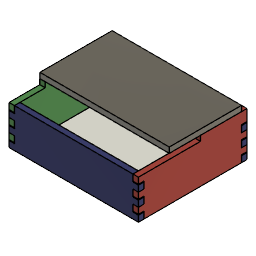
UselessBoxCardboard_v4 (Autodesk Fusion 360 design; units mm, degrees)
Autodesk Fusion 360 part; units mm, degrees
note: some values were not read from the file. Chosen so that the rebuilt part matches the saved one: a direction.
sketch "Sketch1" plane through (0, 0, 0) normal (0, 0, 1) x (1, 0, 0) in component "bottom panel"
  line L0 (0, 0) -> (91, 0)
  line L1 (91, 0) -> (91, 75)
  line L2 (91, 75) -> (0, 75)
  line L3 (0, 75) -> (0, 0)
  dimension "d116" = 75
  dimension "d117" = 91
  constraint horizontal L0
  constraint vertical L1
  constraint horizontal L2
  constraint vertical L3
  constraint coincident L0.start L3.end
  measures "d116" distance of L0.start L2.end
  measures "d117" distance of L1.end L2.end
extrude "Extrude1" add sketch "Sketch1" against normal blind 4.2 makes body 1 in component "bottom panel"
sketch "Sketch1 (2)" plane through (0, 0, 0) normal (0, -1, 0) x (1, 0, 0) in component "front panel"
  line L0 (91, 0) -> (0, 0)
  line L1 (0, 0) -> (0, -4.2)
  line L2 (0, -4.2) -> (91, -4.2)
  line L3 (91, -4.2) -> (91, 0)
  line L4 (0, 30) -> (91, 30)
  line L5 (91, 30) -> (91, 0)
  line L6 (91, 0) -> (0, 0)
  line L7 (0, 0) -> (0, 30)
  line L8 (0, 0) -> (-4.2, 0)
  line L9 (-4.2, 0) -> (-4.2, 5.3)
  line L10 (-4.2, 5.3) -> (0, 5.3)
  line L11 (0, 5.3) -> (0, 0)
  line L12 (45.5, 30) -> (45.5, 0) construction
  line L13 (95.2, 5.3) -> (91, 5.3)
  line L14 (95.2, 0) -> (95.2, 5.3)
  line L15 (91, 0) -> (95.2, 0)
  line L16 (-4.2, 15.3) -> (0, 15.3)
  line L17 (-4.2, 10) -> (-4.2, 15.3)
  line L18 (0, 10) -> (-4.2, 10)
  line L19 (-4.2, 25.3) -> (0, 25.3)
  line L20 (-4.2, 20) -> (-4.2, 25.3)
  line L21 (0, 20) -> (-4.2, 20)
  line L22 (95.2, 15.3) -> (91, 15.3)
  line L23 (95.2, 10) -> (95.2, 15.3)
  line L24 (91, 10) -> (95.2, 10)
  line L25 (95.2, 25.3) -> (91, 25.3)
  line L26 (95.2, 20) -> (95.2, 25.3)
  line L27 (91, 20) -> (95.2, 20)
  dimension "d120" = 30
  dimension "d121" = 5.3
  dimension "d123" = 4.2
  dimension "d126" = 0
  dimension "d127" = 10
  dimension "d130" = 0
  dimension "d131" = 10
  constraint horizontal L4
  constraint vertical L5
  constraint horizontal L6
  constraint vertical L7
  constraint midpoint L0 L6
  constraint equal L0 L6
  constraint horizontal L8
  constraint vertical L9
  constraint horizontal L10
  constraint vertical L11
  constraint midpoint L4 L12.start
  constraint midpoint L6 L12.end
  constraint symmetric L0.end L12 L0.start
  constraint symmetric L8.end L12 L14.start
  constraint symmetric L9.end L12 L13.start
  constraint symmetric L10.end L12 L13.end
  measures "d120" distance of L4.end L0.start
  measures "d121" distance of L8.end L9.end
  measures "d123" distance of L9.end L10.end
extrude "Extrude1'" add sketch "Sketch1 (2)" along normal blind 4.2 separate body contours L0 L4 L5 L6 L7 L11 | L5 L13 L14 L15 | L7 L8 L9 L10 L11 | L5 L22 L23 L24 | L7 L16 L17 L18 | L5 L25 L26 L27 | L7 L19 L20 L21 makes body 2 in component "front panel"
sketch "Sketch1 (3)" plane through (0, 0, 0) normal (-1, 0, 0) x (0, -1, 0) in component "left panel"
  line L0 (0, 0) -> (-75, 0)
  line L1 (-75, 0) -> (-75, -4.2)
  line L2 (-75, -4.2) -> (0, -4.2)
  line L3 (0, -4.2) -> (0, 0)
  line L4 (0, 0) -> (-75, 0)
  line L5 (-75, 0) -> (-75, 30)
  line L6 (-75, 30) -> (0, 30)
  line L7 (0, 30) -> (0, 0)
  line L8 (0, 10) -> (4.2, 10)
  line L9 (4.2, 10) -> (4.2, 4.7)
  line L10 (4.2, 4.7) -> (0, 4.7)
  line L11 (0, 4.7) -> (0, 10)
  line L12 (-37.5, 30) -> (-37.5, 0) construction
  line L13 (-75, 10) -> (-79.2, 10)
  line L14 (-79.2, 10) -> (-79.2, 4.7)
  line L15 (-79.2, 4.7) -> (-75, 4.7)
  line L16 (4.2, 14.7) -> (0, 14.7)
  line L17 (4.2, 20) -> (4.2, 14.7)
  line L18 (0, 20) -> (4.2, 20)
  line L19 (4.2, 24.7) -> (0, 24.7)
  line L20 (4.2, 30) -> (4.2, 24.7)
  line L21 (0, 30) -> (4.2, 30)
  line L22 (-75, 20) -> (-79.2, 20)
  line L23 (-79.2, 20) -> (-79.2, 14.7)
  line L24 (-79.2, 14.7) -> (-75, 14.7)
  line L25 (-75, 30) -> (-79.2, 30)
  line L26 (-79.2, 30) -> (-79.2, 24.7)
  line L27 (-79.2, 24.7) -> (-75, 24.7)
  dimension "d134" = 75
  dimension "d135" = 30
  dimension "d136" = 4.2
  dimension "d137" = 5.3
  dimension "d138" = 4.7
  dimension "d141" = 0
  dimension "d142" = 10
  dimension "d145" = 0
  dimension "d146" = 10
  constraint horizontal L4
  constraint vertical L5
  constraint horizontal L6
  constraint vertical L7
  constraint coincident L0.start L3.end
  constraint horizontal L8
  constraint vertical L9
  constraint horizontal L10
  constraint vertical L11
  constraint coincident L7 L8.start
  constraint midpoint L6 L12.start
  constraint midpoint L4 L12.end
  constraint symmetric L8.start L12 L13.start
  constraint symmetric L8.end L12 L13.end
  constraint symmetric L9.end L12 L14.end
  constraint symmetric L10.end L12 L15.end
  measures "d134" distance of L5.end L6.end
  measures "d135" distance of L0.end L5.end
  measures "d136" distance of L8.start L8.end
  measures "d137" distance of L8.end L9.end
  measures "d138" distance of L0.start L10
extrude "Extrude1''" add sketch "Sketch1 (3)" along normal blind 4.2 separate body contours L0 L4 L5 L6 L7 L11 | L7 L8 L9 L10 L11 | L5 L13 L14 L15 | L7 L16 L17 L18 | L5 L22 L23 L24 | L7 L19 L20 L21 | L5 L25 L26 L27 makes body 3 in component "left panel"
ref_plane "WorkPlane1" through (45.5, 37.5, -2.1) normal (-1, 0, 0) x (0, 1, 0)
ref_plane "WorkPlane2" through (45.5, 37.5, -2.1) normal (0, -1, 0) x (-1, 0, 0)
mirror "MirrorComponent1" about plane through (0, 0, 0) normal (0, 0, 1) of bodies 3 makes body 4 in component "right panel"
mirror "MirrorComponent2" about plane through (0, 0, 0) normal (0, 0, 1) of bodies 2 makes body 5 in component "back panel"
sketch "Sketch15" plane through (0, 0, 30) normal (0, 0, 1) x (-1, 0, 0)
  line L0 (0, 4.2) -> (0, -79.2)
  line L1 (0, -79.2) -> (4.2, -79.2)
  line L2 (4.2, -79.2) -> (4.2, 4.2)
  line L3 (4.2, 4.2) -> (0, 4.2)
  line L4 (0, 4.2) -> (4.2, 4.2)
  line L5 (4.2, 4.2) -> (4.2, -19.45)
  line L6 (4.2, -19.45) -> (0, -19.45)
  line L7 (0, -19.45) -> (0, 4.2)
  dimension "d213" = 4.2
  dimension "d214" = 23.65
  constraint horizontal L4
  constraint vertical L5
  constraint horizontal L6
  constraint vertical L7
  constraint coincident L0.start L3.end
  measures "d213" distance of L0.start L2.end
  measures "d214" distance of L0.start L6.end
extrude "Extrude3" add sketch "Sketch15" along normal blind 4 contours L0 L1 L2 L6 bodies 3 in component "left panel"
extrude "Extrude1'''" add 1 faces at (30.3333, -1.4, -30) along direction (0, 0, -1) blind 4 on bodies 5 bodies 5 in component "back panel"
sketch "Sketch16" plane through (0, 0, 30) normal (0, 0, 1) x (-1, 0, 0)
  line L0 (-91, -79.2) -> (-91, 4.2)
  line L1 (-91, 4.2) -> (-95.2, 4.2)
  line L2 (-95.2, 4.2) -> (-95.2, -79.2)
  line L3 (-95.2, -79.2) -> (-91, -79.2)
  line L4 (-95.2, 4.2) -> (-91, 4.2)
  line L5 (-91, 4.2) -> (-91, -43.45)
  line L6 (-91, -43.45) -> (-95.2, -43.45)
  line L7 (-95.2, -43.45) -> (-95.2, 4.2)
  dimension "d219" = 4.2
  dimension "d220" = 47.65
  constraint horizontal L4
  constraint vertical L5
  constraint horizontal L6
  constraint vertical L7
  constraint coincident L1.end L2.start
  measures "d219" distance of L1.end L0.end
  measures "d220" distance of L1.end L6.end
extrude "Extrude2" add sketch "Sketch16" along normal blind 4 contours L0 L2 L3 L6 sketch seen with x (-1, 0, 0) y (0, 1, 0) z (0, 0, -1) at (91, 0, 0) bodies 4 in component "right panel"
sketch "Sketch2" plane through (0, 0, 34) normal (0, 0, 1) x (-1, 0, 0) in component "lid"
  line L0 (4.2, -19.45) -> (0, -19.45)
  line L1 (0, -19.45) -> (0, -79.2)
  line L2 (0, -79.2) -> (4.2, -79.2)
  line L3 (4.2, -79.2) -> (4.2, -19.45)
  line L4 (4.2, -79.2) -> (-95.2, -79.2)
  line L5 (-95.2, -79.2) -> (-95.2, -19.2)
  line L6 (-95.2, -19.2) -> (4.2, -19.2)
  line L7 (4.2, -19.2) -> (4.2, -79.2)
  dimension "d225" = 99.4
  dimension "d226" = 60
  constraint horizontal L4
  constraint vertical L5
  constraint horizontal L6
  constraint vertical L7
  constraint coincident L2.end L3.start
  measures "d225" distance of L2.end L4.end
  measures "d226" distance of L2.end L6.end
extrude "Extrude2'" add sketch "Sketch2" along normal blind 4.2 separate body makes body 6 in component "lid"
move_face "OffsetFaces1" offset -4.5 1 faces at (28.9333, 19.2, 35.4) on bodies 6 in component "lid"
sketch "Sketch18" plane through (0, 0, 0) normal (0, 0, 1) x (-1, 0, 0)
  line L0 (-95.2, -164.5) -> (4.2, -164.5)
  line L1 (4.2, -164.5) -> (4.2, -109)
  line L2 (4.2, -109) -> (-95.2, -109)
  line L3 (-95.2, -109) -> (-95.2, -164.5)
  line L4 (-91, -85) -> (-95.2, -85)
  line L5 (-95.2, -85) -> (-95.2, -90.3)
  line L6 (-95.2, -90.3) -> (-91, -90.3)
  line L7 (-91, -90.3) -> (-91, -95)
  line L8 (-91, -95) -> (-95.2, -95)
  line L9 (-95.2, -95) -> (-95.2, -100.3)
  line L10 (-95.2, -100.3) -> (-91, -100.3)
  line L11 (-91, -100.3) -> (-91, -109)
  line L12 (-91, -109) -> (0, -109)
  line L13 (0, -109) -> (0, -100.3)
  line L14 (0, -100.3) -> (4.2, -100.3)
  line L15 (4.2, -100.3) -> (4.2, -95)
  line L16 (4.2, -95) -> (0, -95)
  line L17 (0, -95) -> (0, -90.3)
  line L18 (0, -90.3) -> (4.2, -90.3)
  line L19 (4.2, -90.3) -> (4.2, -85)
  line L20 (4.2, -85) -> (0, -85)
  line L21 (0, -85) -> (0, -80.3)
  line L22 (0, -80.3) -> (4.2, -80.3)
  line L23 (4.2, -80.3) -> (4.2, -75)
  line L24 (4.2, -75) -> (-95.2, -75)
  line L25 (-95.2, -75) -> (-95.2, -80.3)
  line L26 (-95.2, -80.3) -> (-91, -80.3)
  line L27 (-91, -80.3) -> (-91, -85)
  line L28 (0, -75) -> (0, 0)
  line L29 (0, 0) -> (-91, 0)
  line L30 (-91, 0) -> (-91, -75)
  line L31 (-91, -75) -> (0, -75)
  line L32 (30, -19.45) -> (30, 4.2)
  line L33 (30, 4.2) -> (24.7, 4.2)
  line L34 (24.7, 4.2) -> (24.7, 0)
  line L35 (24.7, 0) -> (20, 0)
  line L36 (20, 0) -> (20, 4.2)
  line L37 (20, 4.2) -> (14.7, 4.2)
  line L38 (14.7, 4.2) -> (14.7, 0)
  line L39 (14.7, 0) -> (10, 0)
  line L40 (10, 0) -> (10, 4.2)
  line L41 (10, 4.2) -> (4.7, 4.2)
  line L42 (4.7, 4.2) -> (4.7, 0)
  line L43 (4.7, 0) -> (0, 0)
  line L44 (0, 0) -> (0, -75)
  line L45 (0, -75) -> (4.7, -75)
  line L46 (4.7, -75) -> (4.7, -79.2)
  line L47 (4.7, -79.2) -> (10, -79.2)
  line L48 (10, -79.2) -> (10, -75)
  line L49 (10, -75) -> (14.7, -75)
  line L50 (14.7, -75) -> (14.7, -79.2)
  line L51 (14.7, -79.2) -> (20, -79.2)
  line L52 (20, -79.2) -> (20, -75)
  line L53 (20, -75) -> (24.7, -75)
  line L54 (24.7, -75) -> (24.7, -79.2)
  line L55 (24.7, -79.2) -> (34, -79.2)
  line L56 (34, -79.2) -> (34, -19.45)
  line L57 (34, -19.45) -> (30, -19.45)
  line L58 (-95.2, 10) -> (-91, 10)
  line L59 (-91, 10) -> (-91, 5.3)
  line L60 (-91, 5.3) -> (-95.2, 5.3)
  line L61 (-95.2, 5.3) -> (-95.2, 0)
  line L62 (-95.2, 0) -> (4.2, 0)
  line L63 (4.2, 0) -> (4.2, 5.3)
  line L64 (4.2, 5.3) -> (0, 5.3)
  line L65 (0, 5.3) -> (0, 10)
  line L66 (0, 10) -> (4.2, 10)
  line L67 (4.2, 10) -> (4.2, 15.3)
  line L68 (4.2, 15.3) -> (0, 15.3)
  line L69 (0, 15.3) -> (0, 20)
  line L70 (0, 20) -> (4.2, 20)
  line L71 (4.2, 20) -> (4.2, 25.3)
  line L72 (4.2, 25.3) -> (0, 25.3)
  line L73 (0, 25.3) -> (0, 30)
  line L74 (0, 30) -> (-91, 30)
  line L75 (-91, 30) -> (-91, 25.3)
  line L76 (-91, 25.3) -> (-95.2, 25.3)
  line L77 (-95.2, 25.3) -> (-95.2, 20)
  line L78 (-95.2, 20) -> (-91, 20)
  line L79 (-91, 20) -> (-91, 15.3)
  line L80 (-91, 15.3) -> (-95.2, 15.3)
  line L81 (-95.2, 15.3) -> (-95.2, 10)
  line L82 (-125, -79.2) -> (-115.7, -79.2)
  line L83 (-115.7, -79.2) -> (-115.7, -75)
  line L84 (-115.7, -75) -> (-111, -75)
  line L85 (-111, -75) -> (-111, -79.2)
  line L86 (-111, -79.2) -> (-105.7, -79.2)
  line L87 (-105.7, -79.2) -> (-105.7, -75)
  line L88 (-105.7, -75) -> (-101, -75)
  line L89 (-101, -75) -> (-101, -79.2)
  line L90 (-101, -79.2) -> (-95.7, -79.2)
  line L91 (-95.7, -79.2) -> (-95.7, -75)
  line L92 (-95.7, -75) -> (-91, -75)
  line L93 (-91, -75) -> (-91, 0)
  line L94 (-91, 0) -> (-95.7, 0)
  line L95 (-95.7, 0) -> (-95.7, 4.2)
  line L96 (-95.7, 4.2) -> (-101, 4.2)
  line L97 (-101, 4.2) -> (-101, 0)
  line L98 (-101, 0) -> (-105.7, 0)
  line L99 (-105.7, 0) -> (-105.7, 4.2)
  line L100 (-105.7, 4.2) -> (-111, 4.2)
  line L101 (-111, 4.2) -> (-111, 0)
  line L102 (-111, 0) -> (-115.7, 0)
  line L103 (-115.7, 0) -> (-115.7, 4.2)
  line L104 (-115.7, 4.2) -> (-121, 4.2)
  line L105 (-121, 4.2) -> (-121, -43.45)
  line L106 (-121, -43.45) -> (-125, -43.45)
  line L107 (-125, -43.45) -> (-125, -79.2)
component "bottom panel" placed x (1, 0, 0) y (0, 1, 0) z (0, 0, 1) at (0, 0, 0)
component "front panel" placed x (1, 0, 0) y (0, 0, 1) z (0, -1, 0) at (0, 0, 0)
component "left panel" placed x (0, 0, 1) y (0, 1, 0) z (-1, 0, 0) at (0, 0, 0)
component "right panel" placed x (0, 0, 1) y (0, 1, 0) z (-1, 0, 0) at (91, 0, 0)
component "back panel" placed x (1, 0, 0) y (0, 0, 1) z (0, -1, 0) at (0, 75, 0)
component "lid" placed x (1, 0, 0) y (0, -1, 0) z (0, 0, -1) at (0, 188.2, 34)
equation "cardboardThickness = 4.2 mm"
equation "boxFrontLen = 91 mm"
equation "boxHeight = 30 mm"
equation "boxSideLen = 75 mm"
equation "kerf = 0.3 mm"
equation "d116 = boxSideLen"
equation "d117 = boxFrontLen"
equation "d118 = -cardboardThickness"
equation "d120 = boxHeight"
equation "d121 = ( boxHeight / ( numTeeth * 2 ) ) + kerf"
equation "numTeeth = 3"
equation "d123 = cardboardThickness"
equation "d125 = numTeeth"
equation "d127 = boxHeight / ( numTeeth )"
equation "d131 = boxHeight / numTeeth"
equation "d132 = cardboardThickness"
equation "d134 = boxSideLen"
equation "d135 = boxHeight"
equation "d136 = cardboardThickness"
equation "d137 = boxHeight / ( numTeeth * 2 ) + kerf"
equation "d138 = boxHeight / ( numTeeth * 2 ) - kerf"
equation "d142 = boxHeight / numTeeth"
equation "d146 = boxHeight / numTeeth"
equation "d147 = cardboardThickness"
equation "d213 = cardboardThickness"
equation "d219 = cardboardThickness"
equation "d227 = cardboardThickness"
